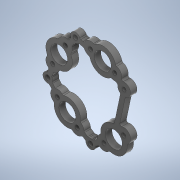
# Autodesk Inventor part: アーム モーターマウントフレーム
Saved by Autodesk Inventor 2020.2 (Build 242310000, 310)
## iProperties
Created: 2020-05-03
Part Number: アーム モーターマウントフレーム
Material: ABS プラスチック
Document SubType Name: Modeling
Designer: mozar
Density: 1.06 g/cm^3
Appearance: 滑らか - 黒
Mass: 3.91189 g
Surface Area: 42.0198 cm^2
Volume: 3.69046 cm^3
Author: mozar
Autodesk Inventor part; units mm, degrees
(part 1 of 2)
ref_plane "YZ Plane" through (0, 0, 0) normal (1, 0, 0) x (0, 1, 0)
ref_plane "XZ Plane" through (0, 0, 0) normal (0, 1, 0) x (-1, 0, 0)
ref_plane "XY Plane" through (0, 0, 0) normal (0, 0, 1) x (1, 0, 0)
sketch "スケッチ1" plane through (0, 0, 0) normal (0, 0, 1) x (1, 0, 0)
  circle A0 centre (-44.5012, 92.4909) radius 1.25
  arc A1 (-69.4548, 57.7196) -> (-69.0181, 56.9729) centre (-68.4582, 57.8015) ccw
  line L0 (-69.0181, 56.9729) -> (-68.4366, 56.58)
  arc A2 (-68.4366, 56.58) -> (-66.8767, 57.4086) centre (-67.8767, 57.4086) ccw
  line L1 (-66.8767, 57.4086) -> (-66.8767, 71.7112)
  arc A3 (-66.8767, 71.7112) -> (-67.5826, 72.667) centre (-67.8767, 71.7112) ccw
  arc A4 (-72.0424, 76.3973) -> (-67.5826, 72.667) centre (-65.3767, 79.8352) ccw
  arc A5 (-72.0424, 76.3973) -> (-73.1078, 76.9232) centre (-72.9311, 75.9389) ccw
  line L2 (-73.1078, 76.9232) -> (-87.1853, 74.3957)
  arc A6 (-87.1853, 74.3957) -> (-87.7252, 72.7139) centre (-87.0086, 73.4114) ccw
  line L3 (-87.7252, 72.7139) -> (-87.2357, 72.211)
  arc A7 (-87.2357, 72.211) -> (-86.4237, 71.9131) centre (-86.5192, 72.9085) ccw
  arc A8 (-83.0085, 70.7089) -> (-86.4237, 71.9131) centre (-86.0131, 67.6327) ccw
  arc A9 (-83.0085, 70.7089) -> (-82.0468, 70.4595) centre (-82.3098, 71.4243) ccw
  arc A10 (-71.659, 61.7707) -> (-82.0468, 70.4595) centre (-79.8767, 62.5) ccw
  arc A11 (-71.659, 61.7707) -> (-71.2436, 60.8681) centre (-70.663, 61.6823) ccw
  arc A12 (-69.4548, 57.7196) -> (-71.2436, 60.8681) centre (-73.7404, 57.3673) ccw
  arc A13 (-69.2468, 101.9882) -> (-69.916, 102.5363) centre (-70.1527, 101.5647) ccw
  line L4 (-69.916, 102.5363) -> (-70.5978, 102.7024)
  arc A14 (-70.5978, 102.7024) -> (-71.772, 101.383) centre (-70.8345, 101.7308) ccw
  line L5 (-71.772, 101.383) -> (-66.7965, 87.9737)
  arc A15 (-66.7965, 87.9737) -> (-65.8023, 87.3231) centre (-65.859, 88.3215) ccw
  arc A16 (-63.8426, 87.1766) -> (-65.8023, 87.3231) centre (-65.3767, 79.8352) ccw
  arc A17 (-63.8426, 87.1766) -> (-62.7626, 87.6721) centre (-63.638, 88.1555) ccw
  line L6 (-62.7626, 87.6721) -> (-60.3455, 92.0492)
  arc A18 (-60.3455, 92.0492) -> (-60.8525, 93.4623) centre (-61.2209, 92.5326) ccw
  arc A19 (-65.771, 98.9569) -> (-60.8525, 93.4623) centre (-57.8128, 101.1319) ccw
  arc A20 (-65.771, 98.9569) -> (-66.4744, 99.6586) centre (-66.7356, 98.6933) ccw
  arc A21 (-69.2468, 101.9882) -> (-66.4744, 99.6586) centre (-65.3514, 103.8094) ccw
  arc A22 (-69.9385, 85.7884) -> (-69.6092, 86.93) centre (-70.5467, 86.5822) ccw
  line L7 (-69.6092, 86.93) -> (-74.5846, 100.3393)
  arc A23 (-74.5846, 100.3393) -> (-76.3353, 100.5735) centre (-75.5222, 99.9915) ccw
  line L8 (-76.3353, 100.5735) -> (-76.7438, 100.0029)
  arc A24 (-76.7438, 100.0029) -> (-76.8935, 99.1509) centre (-75.9306, 99.4208) ccw
  arc A25 (-77.4753, 95.5768) -> (-76.8935, 99.1509) centre (-81.034, 97.9904) ccw
  arc A26 (-77.4753, 95.5768) -> (-77.5508, 94.5861) centre (-76.6477, 95.0154) ccw
  arc A27 (-84.2672, 82.8263) -> (-77.5508, 94.5861) centre (-85.0015, 91.0436) ccw
  arc A28 (-84.2672, 82.8263) -> (-85.0821, 82.2579) centre (-84.1781, 81.8303) ccw
  arc A29 (-87.865, 79.9409) -> (-85.0821, 82.2579) centre (-88.9691, 84.0968) ccw
  arc A30 (-87.865, 79.9409) -> (-88.5227, 79.3791) centre (-87.6082, 78.9744) ccw
  line L9 (-88.5227, 79.3791) -> (-88.8067, 78.7374)
  arc A31 (-88.8067, 78.7374) -> (-87.7155, 77.3484) centre (-87.8922, 78.3327) ccw
  line L10 (-87.7155, 77.3484) -> (-73.638, 79.876)
  arc A32 (-73.638, 79.876) -> (-72.822, 80.7396) centre (-73.8147, 80.8602) ccw
  arc A33 (-69.9385, 85.7884) -> (-72.822, 80.7396) centre (-65.3767, 79.8352) ccw
  arc A34 (13.5891, 109.0089) -> (14.6006, 109.7003) centre (13.6488, 110.0071) ccw
  line L11 (14.6006, 109.7003) -> (22.3119, 133.625)
  arc A35 (22.3119, 133.625) -> (21.598, 134.903) centre (21.3602, 133.9317) ccw
  arc A36 (21.598, 134.903) -> (-12.3137, 125.4554) centre (13.05, 100) ccw
  arc A37 (-12.3137, 125.4554) -> (-11.2534, 123.8119) centre (-11.6078, 124.747) ccw
  arc A38 (-5.288, 118.533) -> (-11.2534, 123.8119) centre (-9.6587, 119.604) ccw
  arc A39 (-5.288, 118.533) -> (-4.9702, 117.5381) centre (-4.3167, 118.295) ccw
  line L12 (-4.9702, 117.5381) -> (6.6814, 107.4795)
  arc A40 (6.6814, 107.4795) -> (7.905, 107.4148) centre (7.3349, 108.2364) ccw
  arc A41 (13.5891, 109.0089) -> (7.905, 107.4148) centre (13.05, 100) ccw
  arc A42 (16.2852, 90.7245) -> (15.1677, 91.227) centre (15.4023, 90.2549) ccw
  arc A43 (12.0966, 91.0255) -> (15.1677, 91.227) centre (13.05, 100) ccw
  arc A44 (12.0966, 91.0255) -> (11.0543, 90.3814) centre (11.9909, 90.0311) ccw
  line L13 (11.0543, 90.3814) -> (-1.3153, 57.3061)
  arc A45 (-1.3153, 57.3061) -> (-0.2632, 55.9625) centre (-0.3787, 56.9558) ccw
  line L14 (-0.2632, 55.9625) -> (26.3316, 59.055)
  arc A46 (26.3316, 59.055) -> (27.2024, 59.8834) centre (26.2161, 60.0483) ccw
  arc A47 (29.5215, 64.3049) -> (27.2024, 59.8834) centre (35.0928, 58.5637) ccw
  arc A48 (29.5215, 64.3049) -> (29.708, 65.4922) centre (28.8251, 65.0226) ccw
  line L15 (29.708, 65.4922) -> (16.2852, 90.7245)
  arc A49 (21.5566, 103.0147) -> (22.5876, 102.3526) centre (22.4992, 103.3487) ccw
  line L16 (22.5876, 102.3526) -> (47.6258, 104.5754)
  arc A50 (47.6258, 104.5754) -> (48.5246, 105.731) centre (47.5374, 105.5715) ccw
  arc A51 (48.5246, 105.731) -> (26.4932, 133.3253) centre (13.05, 100) ccw
  arc A52 (26.4932, 133.3253) -> (25.1673, 132.7046) centre (26.1191, 132.3979) ccw
  line L17 (25.1673, 132.7046) -> (17.4559, 108.78)
  arc A53 (17.4559, 108.78) -> (17.8733, 107.628) centre (18.4077, 108.4732) ccw
  arc A54 (21.5566, 103.0147) -> (17.8733, 107.628) centre (13.05, 100) ccw
  arc A55 (48.9794, 100.608) -> (47.8911, 101.5872) centre (47.9795, 100.5911) ccw
  line L18 (47.8911, 101.5872) -> (22.8529, 99.3644)
  arc A56 (22.8529, 99.3644) -> (21.9546, 98.5311) centre (22.9413, 98.3683) ccw
  arc A57 (19.1416, 93.341) -> (21.9546, 98.5311) centre (13.05, 100) ccw
  arc A58 (19.1416, 93.341) -> (18.9338, 92.1335) centre (19.8166, 92.6031) ccw
  line L19 (18.9338, 92.1335) -> (30.7392, 69.9415)
  arc A59 (30.7392, 69.9415) -> (32.1537, 69.5642) centre (31.622, 70.4111) ccw
  arc A60 (32.1537, 69.5642) -> (48.9794, 100.608) centre (13.05, 100) ccw
  arc A61 (-34.2364, 127.0372) -> (-36.0614, 127.7726) centre (-35.216, 127.2385) ccw
  line L20 (-36.0614, 127.7726) -> (-39.8212, 121.8216)
  arc A62 (-39.8212, 121.8216) -> (-38.4894, 120.4137) centre (-38.9758, 121.2874) ccw
  line L21 (-38.4894, 120.4137) -> (-34.6838, 122.5323)
  arc A63 (-34.6838, 122.5323) -> (-34.1958, 123.6306) centre (-35.1702, 123.406) ccw
  arc A64 (-34.2364, 127.0372) -> (-34.1958, 123.6306) centre (-26.4001, 125.4272) ccw
  arc A65 (5.9328, 94.4506) -> (4.7454, 94.7527) centre (5.1442, 93.8357) ccw
  line L22 (4.7454, 94.7527) -> (-16.5104, 85.5088)
  arc A66 (-16.5104, 85.5088) -> (-17.0899, 84.3844) centre (-16.1116, 84.5918) ccw
  arc A67 (-19.2338, 74.9766) -> (-17.0899, 84.3844) centre (-28.3399, 82) ccw
  arc A68 (-19.2338, 74.9766) -> (-19.1987, 73.7122) centre (-18.4419, 74.3659) ccw
  line L23 (-19.1987, 73.7122) -> (-5.7745, 58.1716)
  arc A69 (-5.7745, 58.1716) -> (-4.0811, 58.475) centre (-5.0177, 58.8253) ccw
  line L24 (-4.0811, 58.475) -> (8.2443, 91.4322)
  arc A70 (8.2443, 91.4322) -> (7.8805, 92.6022) centre (7.3077, 91.7825) ccw
  arc A71 (5.9328, 94.4506) -> (7.8805, 92.6022) centre (13.05, 100) ccw
  arc A72 (4.9636, 104.0076) -> (4.721, 105.2086) centre (4.0676, 104.4516) ccw
  line L25 (4.721, 105.2086) -> (-6.9306, 115.2672)
  arc A73 (-6.9306, 115.2672) -> (-7.9613, 115.4364) centre (-7.5841, 114.5103) ccw
  arc A74 (-9.6102, 115.1042) -> (-7.9613, 115.4364) centre (-9.6587, 119.604) ccw
  arc A75 (-9.6102, 115.1042) -> (-10.495, 114.5492) centre (-9.5994, 114.1043) ccw
  line L26 (-10.495, 114.5492) -> (-21.5476, 92.3011)
  arc A76 (-21.5476, 92.3011) -> (-21.267, 91.0677) centre (-20.652, 91.8562) ccw
  arc A77 (-18.9244, 88.6028) -> (-21.267, 91.0677) centre (-28.3399, 82) ccw
  arc A78 (-18.9244, 88.6028) -> (-17.7068, 88.2599) centre (-18.1056, 89.177) ccw
  line L27 (-17.7068, 88.2599) -> (3.549, 97.5038)
  arc A79 (3.549, 97.5038) -> (4.1377, 98.5784) centre (3.1501, 98.4209) ccw
  arc A80 (4.9636, 104.0076) -> (4.1377, 98.5784) centre (13.05, 100) ccw
  arc A81 (-35.8272, 90.7287) -> (-35.6044, 91.9739) centre (-36.4783, 91.4878) ccw
  line L28 (-35.6044, 91.9739) -> (-45.4441, 109.6631)
  arc A82 (-45.4441, 109.6631) -> (-47.1934, 109.6604) centre (-46.318, 109.177) ccw
  line L29 (-47.1934, 109.6604) -> (-49.9541, 104.6611)
  arc A83 (-49.9541, 104.6611) -> (-50.0229, 103.8484) centre (-49.0787, 104.1777) ccw
  arc A84 (-49.8547, 103.3068) -> (-50.0229, 103.8484) centre (-57.8128, 101.1319) ccw
  arc A85 (-49.8547, 103.3068) -> (-49.1512, 102.6051) centre (-48.89, 103.5704) ccw
  arc A86 (-46.0508, 97.6465) -> (-49.1512, 102.6051) centre (-50.2742, 98.4544) ccw
  arc A87 (-46.0508, 97.6465) -> (-44.9551, 96.465) centre (-45.0686, 97.4586) ccw
  arc A88 (-40.5067, 92.2823) -> (-44.9551, 96.465) centre (-44.5012, 92.4909) ccw
  arc A89 (-40.5067, 92.2823) -> (-40.0525, 91.3914) centre (-39.5081, 92.2301) ccw
  line L30 (-40.0525, 91.3914) -> (-37.7961, 89.9266)
  arc A90 (-37.7961, 89.9266) -> (-36.5387, 90.0642) centre (-37.2516, 90.7654) ccw
  arc A91 (-35.8272, 90.7287) -> (-36.5387, 90.0642) centre (-28.3399, 82) ccw
  arc A92 (-35.3558, 72.8881) -> (-36.6202, 72.8519) centre (-35.9659, 72.0957) ccw
  line L31 (-36.6202, 72.8519) -> (-40.2601, 69.7025)
  arc A93 (-40.2601, 69.7025) -> (-40.5745, 68.6985) centre (-39.6057, 68.9463) ccw
  arc A94 (-42.2436, 64.1319) -> (-40.5745, 68.6985) centre (-44.7404, 67.6327) ccw
  arc A95 (-42.2436, 64.1319) -> (-42.659, 63.2293) centre (-41.663, 63.3177) ccw
  arc A96 (-50.0378, 54.2928) -> (-42.659, 63.2293) centre (-50.8767, 62.5) ccw
  arc A97 (-50.0378, 54.2928) -> (-50.8242, 52.8384) centre (-49.9361, 53.298) ccw
  arc A98 (-50.7048, 52.5865) -> (-50.8242, 52.8384) centre (-54.3767, 51) ccw
  arc A99 (-50.7048, 52.5865) -> (-49.7048, 51.9865) centre (-49.7868, 52.9832) ccw
  arc A100 (-46.9767, 51.2) -> (-49.7048, 51.9865) centre (-49.3767, 48) ccw
  arc A101 (-46.9767, 51.2) -> (-46.3767, 51) centre (-46.3767, 52) ccw
  line L32 (-46.3767, 51) -> (-7.6173, 51)
  arc A102 (-7.6173, 51) -> (-6.7512, 52.5) centre (-7.6173, 52) ccw
  arc A103 (-7.103, 54.5465) -> (-6.7512, 52.5) centre (-4.1532, 54) ccw
  arc A104 (-7.103, 54.5465) -> (-7.3295, 55.3824) centre (-8.0862, 54.7287) ccw
  line L33 (-7.3295, 55.3824) -> (-21.469, 71.7511)
  arc A105 (-21.469, 71.7511) -> (-22.7149, 71.9696) centre (-22.2257, 71.0974) ccw
  arc A106 (-35.3558, 72.8881) -> (-22.7149, 71.9696) centre (-28.3399, 82) ccw
  arc A107 (-43.3166, 71.6902) -> (-42.3312, 71.8776) centre (-42.9855, 72.6338) ccw
  line L34 (-42.3312, 71.8776) -> (-38.5832, 75.1206)
  arc A108 (-38.5832, 75.1206) -> (-38.3657, 76.3667) centre (-39.2375, 75.8768) ccw
  arc A109 (-39.4542, 79.0465) -> (-38.3657, 76.3667) centre (-28.3399, 82) ccw
  arc A110 (-39.4542, 79.0465) -> (-40.479, 79.7879) centre (-40.4207, 78.7896) ccw
  line L35 (-40.479, 79.7879) -> (-57.179, 78.8118)
  arc A111 (-57.179, 78.8118) -> (-58.092, 78.0514) centre (-57.1207, 77.8135) ccw
  arc A112 (-63.1709, 72.667) -> (-58.092, 78.0514) centre (-65.3767, 79.8352) ccw
  arc A113 (-63.1709, 72.667) -> (-63.8767, 71.7112) centre (-62.8767, 71.7112) ccw
  line L36 (-63.8767, 71.7112) -> (-63.8767, 57.4086)
  arc A114 (-63.8767, 57.4086) -> (-62.3169, 56.58) centre (-62.8767, 57.4086) ccw
  line L37 (-62.3169, 56.58) -> (-61.7354, 56.9729)
  arc A115 (-61.7354, 56.9729) -> (-61.2986, 57.7196) centre (-62.2953, 57.8015) ccw
  arc A116 (-59.5099, 60.8681) -> (-61.2986, 57.7196) centre (-57.0131, 57.3673) ccw
  arc A117 (-59.5099, 60.8681) -> (-59.0944, 61.7707) centre (-60.0905, 61.6823) ccw
  arc A118 (-48.7067, 70.4595) -> (-59.0944, 61.7707) centre (-50.8767, 62.5) ccw
  arc A119 (-48.7067, 70.4595) -> (-47.7449, 70.7089) centre (-48.4437, 71.4243) ccw
  arc A120 (-43.3166, 71.6902) -> (-47.7449, 70.7089) centre (-44.7404, 67.6327) ccw
  arc A121 (-24.5231, 117.6505) -> (-25.2874, 116.723) centre (-24.2884, 116.6784) ccw
  line L38 (-25.2874, 116.723) -> (-26.2949, 94.1683)
  arc A122 (-26.2949, 94.1683) -> (-25.5394, 93.1538) centre (-25.2959, 94.1237) ccw
  arc A123 (-25.3867, 93.1143) -> (-25.5394, 93.1538) centre (-28.3399, 82) ccw
  arc A124 (-25.3867, 93.1143) -> (-24.2343, 93.6359) centre (-25.1298, 94.0808) ccw
  line L39 (-24.2343, 93.6359) -> (-13.1817, 115.8839)
  arc A125 (-13.1817, 115.8839) -> (-13.2739, 116.9243) centre (-14.0773, 116.3288) ccw
  arc A126 (-14.1165, 118.9889) -> (-13.2739, 116.9243) centre (-9.6587, 119.604) ccw
  arc A127 (-14.1165, 118.9889) -> (-14.7786, 119.7967) centre (-15.1071, 118.8522) ccw
  line L40 (-14.7786, 119.7967) -> (-18.727, 121.17)
  arc A128 (-18.727, 121.17) -> (-19.8716, 120.8035) centre (-19.0555, 120.2256) ccw
  arc A129 (-24.5231, 117.6505) -> (-19.8716, 120.8035) centre (-26.4001, 125.4272) ccw
  arc A130 (-30.1348, 93.3591) -> (-29.2919, 94.3022) centre (-30.2909, 94.3468) ccw
  line L41 (-29.2919, 94.3022) -> (-28.2844, 116.8569)
  arc A131 (-28.2844, 116.8569) -> (-28.9631, 117.8488) centre (-29.2834, 116.9015) ccw
  arc A132 (-32.0339, 119.7474) -> (-28.9631, 117.8488) centre (-26.4001, 125.4272) ccw
  arc A133 (-32.0339, 119.7474) -> (-33.2246, 119.9111) centre (-32.7382, 119.0374) ccw
  line L42 (-33.2246, 119.9111) -> (-42.8681, 114.5425)
  arc A134 (-42.8681, 114.5425) -> (-43.3678, 113.8351) centre (-42.3817, 113.6687) ccw
  arc A135 (-43.549, 113.1991) -> (-43.3678, 113.8351) centre (-46.326, 114.3342) ccw
  arc A136 (-43.549, 113.1991) -> (-43.4972, 112.3347) centre (-42.6234, 112.8208) ccw
  line L43 (-43.4972, 112.3347) -> (-32.9827, 93.4322)
  arc A137 (-32.9827, 93.4322) -> (-31.8073, 92.9648) centre (-32.1088, 93.9183) ccw
  arc A138 (-30.1348, 93.3591) -> (-31.8073, 92.9648) centre (-28.3399, 82) ccw
  arc A139 (-39.0433, 86.2058) -> (-39.4295, 87.4103) centre (-39.974, 86.5715) ccw
  line L44 (-39.4295, 87.4103) -> (-41.686, 88.875)
  arc A140 (-41.686, 88.875) -> (-42.6846, 88.9272) centre (-42.2304, 88.0363) ccw
  arc A141 (-48.4958, 92.6994) -> (-42.6846, 88.9272) centre (-44.5012, 92.4909) ccw
  arc A142 (-48.4958, 92.6994) -> (-48.95, 93.5904) centre (-49.4944, 92.7516) ccw
  line L45 (-48.95, 93.5904) -> (-49.574, 93.9954)
  arc A143 (-49.574, 93.9954) -> (-50.1478, 94.1562) centre (-50.1185, 93.1567) ccw
  arc A144 (-52.021, 94.5252) -> (-50.1478, 94.1562) centre (-50.2742, 98.4544) ccw
  arc A145 (-52.021, 94.5252) -> (-53.0094, 94.4244) centre (-52.4272, 93.6114) ccw
  arc A146 (-55.9627, 93.092) -> (-53.0094, 94.4244) centre (-57.8128, 101.1319) ccw
  arc A147 (-55.9627, 93.092) -> (-56.6139, 92.6009) centre (-55.7385, 92.1174) ccw
  line L46 (-56.6139, 92.6009) -> (-60.1364, 86.2219)
  arc A148 (-60.1364, 86.2219) -> (-59.9805, 85.044) centre (-59.261, 85.7385) ccw
  arc A149 (-58.3494, 82.4556) -> (-59.9805, 85.044) centre (-65.3767, 79.8352) ccw
  arc A150 (-58.3494, 82.4556) -> (-57.3541, 81.8067) centre (-57.4124, 82.805) ccw
  line L47 (-57.3541, 81.8067) -> (-40.6541, 82.7828)
  arc A151 (-40.6541, 82.7828) -> (-39.7226, 83.6386) centre (-40.7124, 83.7811) ccw
  arc A152 (-39.0433, 86.2058) -> (-39.7226, 83.6386) centre (-28.3399, 82) ccw
  arc A153 (-76.6906, 54.239) -> (-78.3767, 53.5115) centre (-77.3767, 53.5115) ccw
  line L48 (-78.3767, 53.5115) -> (-78.3767, 52)
  arc A154 (-78.3767, 52) -> (-77.3767, 51) centre (-77.3767, 52) ccw
  line L49 (-77.3767, 51) -> (-69.3767, 51)
  arc A155 (-69.3767, 51) -> (-68.7767, 51.2) centre (-69.3767, 52) ccw
  arc A156 (-68.7327, 51.2326) -> (-68.7767, 51.2) centre (-66.3767, 48) ccw
  arc A157 (-68.7327, 51.2326) -> (-68.3354, 52.206) centre (-69.3217, 52.0407) ccw
  arc A158 (-68.3669, 52.4596) -> (-68.3354, 52.206) centre (-65.3767, 52.702) ccw
  arc A159 (-68.3669, 52.4596) -> (-68.8038, 53.2074) centre (-69.3637, 52.3788) ccw
  line L50 (-68.8038, 53.2074) -> (-69.9585, 53.9877)
  arc A160 (-69.9585, 53.9877) -> (-71.1263, 53.9531) centre (-70.5184, 53.1591) ccw
  arc A161 (-76.6906, 54.239) -> (-71.1263, 53.9531) centre (-73.7404, 57.3673) ccw
  arc A162 (23.6969, 52.5865) -> (24.6969, 51.9865) centre (24.6149, 52.9832) ccw
  arc A163 (27.425, 51.2) -> (24.6969, 51.9865) centre (25.025, 48) ccw
  arc A164 (27.425, 51.2) -> (28.025, 51) centre (28.025, 52) ccw
  line L51 (28.025, 51) -> (28.935, 51)
  arc A165 (28.935, 51) -> (29.6192, 52.7293) centre (28.935, 52) ccw
  arc A166 (27.7157, 55.4687) -> (29.6192, 52.7293) centre (35.0928, 58.5637) ccw
  arc A167 (27.7157, 55.4687) -> (26.6781, 56.0751) centre (26.7936, 55.0818) ccw
  line L52 (26.6781, 56.0751) -> (23.2864, 55.6807)
  arc A168 (23.2864, 55.6807) -> (22.7265, 53.9499) centre (23.4019, 54.6874) ccw
  arc A169 (23.6969, 52.5865) -> (22.7265, 53.9499) centre (20.025, 51) ccw
  arc A170 (5.025, 51) -> (5.625, 51.2) centre (5.025, 52) ccw
  arc A171 (8.3531, 51.9865) -> (5.625, 51.2) centre (8.025, 48) ccw
  arc A172 (8.3531, 51.9865) -> (7.8023, 53.8801) centre (7.9178, 52.8868) ccw
  line L53 (7.8023, 53.8801) -> (0.176, 52.9933)
  arc A173 (0.176, 52.9933) -> (0.2915, 51) centre (0.2915, 52) ccw
  line L54 (0.2915, 51) -> (5.025, 51)
  arc A174 (-48.3767, 48) -> (-50.3767, 48) centre (-49.3767, 48) ccw
  line L55 (-50.3767, 48) -> (-50.3767, 45)
  line L56 (-50.3767, 45) -> (-65.3767, 45)
  line L57 (-65.3767, 45) -> (-65.3767, 48)
  arc A175 (-65.3767, 48) -> (-67.3767, 48) centre (-66.3767, 48) ccw
  line L58 (-67.3767, 48) -> (-81.3767, 48)
  line L59 (-81.3767, 48) -> (-81.3767, 53.5942)
  arc A176 (-81.3767, 53.5942) -> (-82.1065, 54.557) centre (-82.3767, 53.5942) ccw
  arc A177 (-88.0944, 63.2293) -> (-82.1065, 54.557) centre (-79.8767, 62.5) ccw
  arc A178 (-88.0944, 63.2293) -> (-88.5099, 64.1319) centre (-89.0905, 63.3177) ccw
  arc A179 (-89.8355, 69.6024) -> (-88.5099, 64.1319) centre (-86.0131, 67.6327) ccw
  arc A180 (-89.8355, 69.6024) -> (-90.0078, 70.7579) centre (-90.7244, 70.0604) ccw
  line L60 (-90.0078, 70.7579) -> (-90.9798, 71.7565)
  arc A181 (-90.9798, 71.7565) -> (-91.7931, 72.0544) centre (-91.6964, 71.059) ccw
  arc A182 (-92.8499, 77.9406) -> (-91.7931, 72.0544) centre (-92.0829, 75.0403) ccw
  arc A183 (-92.8499, 77.9406) -> (-92.1911, 78.5027) centre (-93.1056, 78.9074) ccw
  line L61 (-92.1911, 78.5027) -> (-91.6272, 79.7771)
  arc A184 (-91.6272, 79.7771) -> (-91.8676, 80.9205) centre (-92.5416, 80.1818) ccw
  arc A185 (-92.5278, 86.5104) -> (-91.8676, 80.9205) centre (-88.9691, 84.0968) ccw
  arc A186 (-92.5278, 86.5104) -> (-92.4523, 87.5011) centre (-93.3554, 87.0717) ccw
  arc A187 (-85.7359, 99.2608) -> (-92.4523, 87.5011) centre (-85.0015, 91.0436) ccw
  arc A188 (-85.7359, 99.2608) -> (-84.921, 99.8292) centre (-85.8249, 100.2569) ccw
  arc A189 (-79.7708, 102.1007) -> (-84.921, 99.8292) centre (-81.034, 97.9904) ccw
  arc A190 (-79.7708, 102.1007) -> (-78.6639, 102.4745) centre (-79.4771, 103.0566) ccw
  line L62 (-78.6639, 102.4745) -> (-77.8528, 103.6077)
  arc A191 (-77.8528, 103.6077) -> (-77.7034, 104.4608) centre (-78.6659, 104.1898) ccw
  arc A192 (-72.0965, 106.5412) -> (-77.7034, 104.4608) centre (-74.8156, 105.2737) ccw
  arc A193 (-72.0965, 106.5412) -> (-71.4268, 105.9921) centre (-71.1901, 106.9637) ccw
  line L63 (-71.4268, 105.9921) -> (-70.0728, 105.6623)
  arc A194 (-70.0728, 105.6623) -> (-68.99, 106.1009) centre (-69.8361, 106.6338) ccw
  arc A195 (-63.6047, 107.7386) -> (-68.99, 106.1009) centre (-65.3514, 103.8094) ccw
  arc A196 (-63.6047, 107.7386) -> (-62.6162, 107.8393) centre (-63.1984, 108.6523) ccw
  arc A197 (-52.9408, 107.7896) -> (-62.6162, 107.8393) centre (-57.8128, 101.1319) ccw
  arc A198 (-52.9408, 107.7896) -> (-51.4748, 108.1132) centre (-52.3502, 108.5966) ccw
  line L64 (-51.4748, 108.1132) -> (-49.1485, 112.3259)
  arc A199 (-49.1485, 112.3259) -> (-49.0994, 113.1906) centre (-50.0239, 112.8093) ccw
  arc A200 (-46.6603, 117.3156) -> (-49.0994, 113.1906) centre (-46.326, 114.3342) ccw
  arc A201 (-46.6603, 117.3156) -> (-45.9263, 117.7752) centre (-46.7717, 118.3093) ccw
  line L65 (-45.9263, 117.7752) -> (-37.8629, 130.5378)
  arc A202 (-37.8629, 130.5378) -> (-37.763, 131.3981) centre (-38.7083, 131.0719) ccw
  arc A203 (-31.9852, 132.9642) -> (-37.763, 131.3981) centre (-34.927, 132.3764) ccw
  arc A204 (-31.9852, 132.9642) -> (-30.493, 132.3009) centre (-31.0046, 133.1602) ccw
  arc A205 (-18.408, 125.7823) -> (-30.493, 132.3009) centre (-26.4001, 125.4272) ccw
  arc A206 (-18.408, 125.7823) -> (-16.6463, 125.18) centre (-17.409, 125.8267) ccw
  arc A207 (35.6612, 68.3041) -> (-16.6463, 125.18) centre (13.05, 100) ccw
  arc A208 (35.6612, 68.3041) -> (36.1143, 66.4982) centre (36.242, 67.49) ccw
  arc A209 (42.206, 54.9028) -> (36.1143, 66.4982) centre (35.0928, 58.5637) ccw
  arc A210 (42.206, 54.9028) -> (42.9601, 53.4544) centre (43.0951, 54.4452) ccw
  arc A211 (41.0782, 47.8705) -> (42.9601, 53.4544) centre (42.5549, 50.4818) ccw
  arc A212 (41.0782, 47.8705) -> (40.586, 48) centre (40.586, 47) ccw
  line L66 (40.586, 48) -> (26.025, 48)
  arc A213 (26.025, 48) -> (24.025, 48) centre (25.025, 48) ccw
  line L67 (24.025, 48) -> (24.025, 45)
  line L68 (24.025, 45) -> (9.025, 45)
  line L69 (9.025, 45) -> (9.025, 48)
  arc A214 (9.025, 48) -> (7.025, 48) centre (8.025, 48) ccw
  line L70 (7.025, 48) -> (-48.3767, 48)
  arc A215 (-55.3767, 48) -> (-53.3767, 48) centre (-54.3767, 48) ccw
  line L71 (-53.3767, 48) -> (-53.3767, 51)
  arc A216 (-53.3767, 51) -> (-55.3767, 51) centre (-54.3767, 51) ccw
  line L72 (-55.3767, 51) -> (-60.3767, 51)
  arc A217 (-60.3767, 51) -> (-62.3767, 51) centre (-61.3767, 51) ccw
  line L73 (-62.3767, 51) -> (-62.3767, 48)
  arc A218 (-62.3767, 48) -> (-60.3767, 48) centre (-61.3767, 48) ccw
  line L74 (-60.3767, 48) -> (-55.3767, 48)
  arc A219 (12.025, 48) -> (14.025, 48) centre (13.025, 48) ccw
  line L75 (14.025, 48) -> (19.025, 48)
  arc A220 (19.025, 48) -> (21.025, 48) centre (20.025, 48) ccw
  line L76 (21.025, 48) -> (21.025, 51)
  arc A221 (21.025, 51) -> (19.025, 51) centre (20.025, 51) ccw
  line L77 (19.025, 51) -> (14.025, 51)
  arc A222 (14.025, 51) -> (12.025, 51) centre (13.025, 51) ccw
  line L78 (12.025, 51) -> (12.025, 48)
  circle A223 centre (-4.1532, 54) radius 1.5
  circle A224 centre (-46.326, 114.3342) radius 1.5
  circle A225 centre (-34.927, 132.3764) radius 1.5
  circle A226 centre (42.5549, 50.4818) radius 1.5
  circle A227 centre (-26.4001, 125.4272) radius 4
  circle A228 centre (35.0928, 58.5637) radius 4
  circle A229 centre (-74.8156, 105.2737) radius 1.5
  circle A230 centre (-65.3767, 52.702) radius 1.5
  circle A231 centre (-44.7404, 67.6327) radius 1.3
  circle A232 centre (-57.0131, 57.3673) radius 1.3
  circle A233 centre (-50.8767, 62.5) radius 5.25
  circle A234 centre (-92.0829, 75.0403) radius 1.5
  circle A235 centre (-65.3767, 79.8352) radius 4.5
  circle A236 centre (-28.3399, 82) radius 7.5
  circle A237 centre (-73.7404, 57.3673) radius 1.3
  circle A238 centre (-86.0131, 67.6327) radius 1.3
  circle A239 centre (-79.8767, 62.5) radius 5.25
  circle A240 centre (-65.3514, 103.8094) radius 1.3
  circle A241 centre (-50.2742, 98.4544) radius 1.3
  circle A242 centre (-57.8128, 101.1319) radius 5.25
  circle A243 centre (-9.6587, 119.604) radius 1.5
  circle A244 centre (13.05, 100) radius 4.025
  circle A245 centre (-88.9691, 84.0968) radius 1.3
  circle A246 centre (-81.034, 97.9904) radius 1.3
  circle A247 centre (-85.0015, 91.0436) radius 5.25
  line L79 (-50.8767, 62.5) -> (-44.5012, 92.4909) construction
  line L80 (-49.4095, 62.1881) -> (-43.034, 92.179)
  line L81 (-45.9685, 92.8028) -> (-52.344, 62.8119)
  arc A248 (-52.344, 62.8119) -> (-49.4095, 62.1881) centre (-50.8767, 62.5) ccw
  arc A249 (-43.034, 92.179) -> (-45.9685, 92.8028) centre (-44.5012, 92.4909) ccw
  circle A250 centre (-65.3767, 79.8352) radius 7.5
  circle A251 centre (-57.8128, 101.1319) radius 8.25
  line L82 (-65.3767, 79.8352) -> (-44.5012, 92.4909) construction
  line L83 (-64.5991, 78.5525) -> (-43.7236, 91.2082)
  line L84 (-45.2789, 93.7736) -> (-66.1544, 81.1179)
  arc A252 (-66.1544, 81.1179) -> (-64.5991, 78.5525) centre (-65.3767, 79.8352) ccw
  arc A253 (-43.7236, 91.2082) -> (-45.2789, 93.7736) centre (-44.5012, 92.4909) ccw
  circle A254 centre (-79.8767, 62.5) radius 8.25
  circle A255 centre (-65.3767, 52.702) radius 3
  line L85 (-65.3767, 52.702) -> (-50.8767, 62.5) construction
  line L86 (-64.5369, 51.4592) -> (-50.0369, 61.2571)
  line L87 (-51.7166, 63.7429) -> (-66.2166, 53.9449)
  arc A256 (-66.2166, 53.9449) -> (-64.5369, 51.4592) centre (-65.3767, 52.702) ccw
  arc A257 (-50.0369, 61.2571) -> (-51.7166, 63.7429) centre (-50.8767, 62.5) ccw
  circle A258 centre (-57.0131, 57.3673) radius 4.3
  circle A259 centre (-50.8767, 62.5) radius 8.25
  circle A260 centre (-44.7404, 67.6327) radius 4.3
  circle A261 centre (-44.5012, 92.4909) radius 4
  circle A262 centre (-73.7404, 57.3673) radius 4.3
  point P0 (0, 0)
  point P1 (0, 0)
  point P2 (-47.689, 77.4954)
  point P3 (-54.939, 86.163)
  point P4 (-58.1267, 57.601)
  point P5 (-59.8705, 84.9275)
  point P6 (-59.9805, 85.044)
  point P7 (-48.4498, 91.8512)
  point P8 (-58.3104, 82.365)
  point P9 (-46.8945, 89.2858)
  point P10 (-46.7395, 89.1757)
  point P11 (-50.6571, 70.7471)
  point P12 (-59.0189, 61.1708)
  point P13 (-61.3117, 57.2592)
  point P14 (-64.0639, 55.3995)
  point P15 (-62.3842, 52.9138)
  point P16 (-60.1485, 54.4246)
  point P17 (-53.6239, 54.7208)
  point P18 (-42.659, 63.2293)
  point P19 (-42.7345, 63.8292)
  point P20 (-47.5624, 70.8772)
  point P21 (-43.8051, 88.5519)
  point P22 (-42.6846, 88.9272)
  point P23 (-50.0229, 103.8484)
  point P24 (-74.4553, 56.2815)
  point P25 (-72.798, 58.2628)
  point P26 (-67.5826, 72.667)
  point P27 (-58.092, 78.0514)
  point P28 (-77.1295, 54.7208)
  point P29 (-67.5826, 72.667)
  point P30 (-71.7345, 61.1708)
  dimension "d0" = 3
  dimension "d1" = 3
  dimension "d2" = 3
  constraints: 456 point on circle, 255 centre point, 182 end point, 13 horizontal, 12 tangent, 12 vertical, 9 coincident, 3 concentric, 3 midpoint, 3 parallel, 877 other
  measures "d0" diameter of A249
  measures "d1" diameter of A253
  measures "d2" diameter of A257
extrude "押し出し1" add sketch "スケッチ1" against normal blind 4 contours A262 A161 A254 A237 A12 | A1 L0 A2 L1 A3 A250 A113 L36 A114 L87 A255 A159 L50 A160 A262 | A254 A262 A239 A177 A238 A10 | A254 A237 A262 A239 | A254 A238 A178 A179 A180 L60 A181 A182 A183 L61 A184 A185 A186 A187 A188 A189 A190 L62 A191 A192 A193 L63 A194 A195 A196 A251 A240 A20 A21 A13 L4 A14 L5 A15 A250 A22 L7 A23 L8 A24 A25 A26 A27 A28 A29 A30 L9 A31 L10 A32 A5 L2 A6 L3 A7 A8 A9 | A4 A250 A33 A16 A149 L84 A235 L83 A112 | A255 L87 A230 L86 A158 | L87 L37 A258 L86 A255 | A255 L86 A230 L87 | A258 L87 A259 A232 L86 | L86 A232 A259 A258 | L81 L47 L80 L35 | L35 L80 A120 A119 A118 L81 | L83 A235 L84 A149 A150 | A150 A149 L84 A141 L83 | A258 A116 A259 L87 | A259 A232 L86 A233 A258 | A258 A233 A260 A259 A96 | L81 A141 L80 L47 | L81 A233 A258 A259 A118 | A118 A259 A260 A233 L81 | L83 L81 A141 | A141 L84 A249 L81 L83 | A259 L87 A233 L86 A232 | A259 A258 A233 L87 | L80 A259 A260 A120 | A120 A260 A94 A259 A231 L80 | L81 L83 A253 L80 A141 | A119 A260 A259 | A141 A261 A88 L80 A249 L84 | L81 A249 A253 L83 | A259 A231 A260 A233 L80 | L80 A233 A260 A259 | A142 L45 A143 A144 A145 A251 A241 A85 A86 A87 A261 | A19 A251 A240 A197 A84 A241 A146
fillet "フィレット1" radius 1 15 edges at (-46.8945, 89.2858, -2) (-46.7395, 89.1757, -2) (-50.6571, 70.7471, -2) (-59.0189, 61.1708, -2) (-61.3117, 57.2592, -2) (-71.7345, 61.1708, -2) (-62.3842, 52.9138, -2) (-77.1295, 54.7208, -2) (-60.1485, 54.4246, -2) (-53.6239, 54.7208, -2) (-42.7345, 63.8292, -2) (-47.5624, 70.8772, -2) (-43.8051, 88.5519, -2) (-59.8705, 84.9275, -2) (-48.4498, 91.8512, -2)
sketch "スケッチ2" plane through (0, 0, 0) normal (0, 0, 1) x (1, 0, 0)
  arc A0 (-83.0085, 70.7089) -> (-82.0468, 70.4595) centre (-82.3098, 71.4243) ccw projected
  arc A1 (-71.659, 61.7707) -> (-82.0468, 70.4595) centre (-79.8767, 62.5) ccw projected
  arc A2 (-71.659, 61.7707) -> (-71.2436, 60.8681) centre (-70.663, 61.6823) ccw projected
  arc A3 (-69.4548, 57.7196) -> (-71.2436, 60.8681) centre (-73.7404, 57.3673) ccw projected
  arc A4 (-69.4548, 57.7196) -> (-69.0181, 56.9729) centre (-68.4582, 57.8015) ccw projected
  line L0 (-69.0181, 56.9729) -> (-68.4366, 56.58) projected
  arc A5 (-68.4366, 56.58) -> (-66.8767, 57.4086) centre (-67.8767, 57.4086) ccw projected
  line L1 (-66.8767, 57.4086) -> (-66.8767, 71.7112) projected
  arc A6 (-66.8767, 71.7112) -> (-67.5826, 72.667) centre (-67.8767, 71.7112) ccw projected
  arc A7 (-72.0424, 76.3973) -> (-67.5826, 72.667) centre (-65.3767, 79.8352) ccw projected
  arc A8 (-72.0424, 76.3973) -> (-73.1078, 76.9232) centre (-72.9311, 75.9389) ccw projected
  line L2 (-73.1078, 76.9232) -> (-87.1853, 74.3957) projected
  arc A9 (-87.1853, 74.3957) -> (-87.7252, 72.7139) centre (-87.0086, 73.4114) ccw projected
  line L3 (-87.7252, 72.7139) -> (-87.2357, 72.211) projected
  arc A10 (-87.2357, 72.211) -> (-86.4237, 71.9131) centre (-86.5192, 72.9085) ccw projected
  arc A11 (-83.0085, 70.7089) -> (-86.4237, 71.9131) centre (-86.0131, 67.6327) ccw projected
  circle A12 centre (-73.7404, 57.3673) radius 1.3 projected
  circle A13 centre (-65.3767, 79.8352) radius 4.5 projected
  circle A14 centre (-74.8156, 105.2737) radius 1.5 projected
  circle A15 centre (-92.0829, 75.0403) radius 1.5 projected
  circle A16 centre (-85.0015, 91.0436) radius 5.25 projected
  circle A17 centre (-88.9691, 84.0968) radius 1.3 projected
  circle A18 centre (-81.034, 97.9904) radius 1.3 projected
  circle A19 centre (-65.3514, 103.8094) radius 1.3 projected
  circle A20 centre (-50.2742, 98.4544) radius 1.3 projected
  circle A21 centre (-57.8128, 101.1319) radius 5.25 projected
  circle A22 centre (-86.0131, 67.6327) radius 1.3 projected
  circle A23 centre (-79.8767, 62.5) radius 5.25 projected
  arc A24 (-73.638, 79.876) -> (-72.822, 80.7396) centre (-73.8147, 80.8602) ccw projected
  arc A25 (-69.9385, 85.7884) -> (-72.822, 80.7396) centre (-65.3767, 79.8352) ccw projected
  arc A26 (-69.9385, 85.7884) -> (-69.6092, 86.93) centre (-70.5467, 86.5822) ccw projected
  line L4 (-69.6092, 86.93) -> (-74.5846, 100.3393) projected
  arc A27 (-74.5846, 100.3393) -> (-76.3353, 100.5735) centre (-75.5222, 99.9915) ccw projected
  line L5 (-76.3353, 100.5735) -> (-76.7438, 100.0029) projected
  arc A28 (-76.7438, 100.0029) -> (-76.8935, 99.1509) centre (-75.9306, 99.4208) ccw projected
  arc A29 (-77.4753, 95.5768) -> (-76.8935, 99.1509) centre (-81.034, 97.9904) ccw projected
  arc A30 (-77.4753, 95.5768) -> (-77.5508, 94.5861) centre (-76.6477, 95.0154) ccw projected
  arc A31 (-84.2672, 82.8263) -> (-77.5508, 94.5861) centre (-85.0015, 91.0436) ccw projected
  arc A32 (-84.2672, 82.8263) -> (-85.0821, 82.2579) centre (-84.1781, 81.8303) ccw projected
  arc A33 (-87.865, 79.9409) -> (-85.0821, 82.2579) centre (-88.9691, 84.0968) ccw projected
  arc A34 (-87.865, 79.9409) -> (-88.5227, 79.3791) centre (-87.6082, 78.9744) ccw projected
  line L6 (-88.5227, 79.3791) -> (-88.8067, 78.7374) projected
  arc A35 (-88.8067, 78.7374) -> (-87.7155, 77.3484) centre (-87.8922, 78.3327) ccw projected
  line L7 (-87.7155, 77.3484) -> (-73.638, 79.876) projected
  circle A36 centre (-44.5012, 92.4909) radius 1.25 projected
  arc A37 (-69.2468, 101.9882) -> (-66.4744, 99.6586) centre (-65.3514, 103.8094) ccw projected
  arc A38 (-69.2468, 101.9882) -> (-69.916, 102.5363) centre (-70.1527, 101.5647) ccw projected
  line L8 (-69.916, 102.5363) -> (-70.5978, 102.7024) projected
  arc A39 (-70.5978, 102.7024) -> (-71.772, 101.383) centre (-70.8345, 101.7308) ccw projected
  line L9 (-71.772, 101.383) -> (-66.7965, 87.9737) projected
  arc A40 (-66.7965, 87.9737) -> (-65.8023, 87.3231) centre (-65.859, 88.3215) ccw projected
  arc A41 (-60.3905, 85.4377) -> (-65.8023, 87.3231) centre (-65.3767, 79.8352) ccw projected
  arc A42 (-60.3905, 85.4377) -> (-59.2073, 85.3296) centre (-59.7257, 86.1847) ccw projected
  line L10 (-59.2073, 85.3296) -> (-48.9817, 91.5288) projected
  arc A43 (-48.9817, 91.5288) -> (-48.5003, 92.4053) centre (-49.5001, 92.3839) ccw projected
  arc A44 (-48.4958, 92.6994) -> (-48.5003, 92.4053) centre (-44.5012, 92.4909) ccw projected
  arc A45 (-48.4958, 92.6994) -> (-48.95, 93.5904) centre (-49.4944, 92.7516) ccw projected
  line L11 (-48.95, 93.5904) -> (-49.574, 93.9954) projected
  arc A46 (-49.574, 93.9954) -> (-50.1478, 94.1562) centre (-50.1185, 93.1567) ccw projected
  arc A47 (-52.021, 94.5252) -> (-50.1478, 94.1562) centre (-50.2742, 98.4544) ccw projected
  arc A48 (-52.021, 94.5252) -> (-53.0094, 94.4244) centre (-52.4272, 93.6114) ccw projected
  arc A49 (-65.771, 98.9569) -> (-53.0094, 94.4244) centre (-57.8128, 101.1319) ccw projected
  arc A50 (-65.771, 98.9569) -> (-66.4744, 99.6586) centre (-66.7356, 98.6933) ccw projected
  circle A51 centre (-65.3767, 52.702) radius 1.5 projected
  circle A52 centre (-57.0131, 57.3673) radius 1.3 projected
  circle A53 centre (-50.8767, 62.5) radius 5.25 projected
  circle A54 centre (-44.7404, 67.6327) radius 1.3 projected
  line L12 (-63.8767, 71.7112) -> (-63.8767, 57.4086) projected
  arc A55 (-63.8767, 57.4086) -> (-62.3169, 56.58) centre (-62.8767, 57.4086) ccw projected
  line L13 (-62.3169, 56.58) -> (-61.7354, 56.9729) projected
  arc A56 (-61.7354, 56.9729) -> (-61.2986, 57.7196) centre (-62.2953, 57.8015) ccw projected
  arc A57 (-59.5099, 60.8681) -> (-61.2986, 57.7196) centre (-57.0131, 57.3673) ccw projected
  arc A58 (-59.5099, 60.8681) -> (-59.0944, 61.7707) centre (-60.0905, 61.6823) ccw projected
  arc A59 (-51.4061, 70.733) -> (-59.0944, 61.7707) centre (-50.8767, 62.5) ccw projected
  arc A60 (-51.4061, 70.733) -> (-50.4921, 71.523) centre (-51.4703, 71.7309) ccw projected
  line L14 (-50.4921, 71.523) -> (-47.1705, 87.1482) projected
  arc A61 (-47.1705, 87.1482) -> (-48.6671, 88.2112) centre (-48.1487, 87.3561) ccw projected
  line L15 (-48.6671, 88.2112) -> (-58.3104, 82.365) projected
  arc A62 (-58.3494, 82.4556) -> (-58.3104, 82.365) centre (-57.4124, 82.805) ccw projected
  arc A63 (-63.1709, 72.667) -> (-58.3494, 82.4556) centre (-65.3767, 79.8352) ccw projected
  arc A64 (-63.1709, 72.667) -> (-63.8767, 71.7112) centre (-62.8767, 71.7112) ccw projected
  arc A65 (-69.9585, 53.9877) -> (-71.1263, 53.9531) centre (-70.5184, 53.1591) ccw projected
  arc A66 (-76.7449, 54.2911) -> (-71.1263, 53.9531) centre (-73.7404, 57.3673) ccw projected
  arc A67 (-76.7449, 54.2911) -> (-77.7067, 54.5405) centre (-77.4437, 53.5757) ccw projected
  arc A68 (-88.0944, 63.2293) -> (-77.7067, 54.5405) centre (-79.8767, 62.5) ccw projected
  arc A69 (-88.0944, 63.2293) -> (-88.5099, 64.1319) centre (-89.0905, 63.3177) ccw projected
  arc A70 (-89.8355, 69.6024) -> (-88.5099, 64.1319) centre (-86.0131, 67.6327) ccw projected
  arc A71 (-89.8355, 69.6024) -> (-90.0078, 70.7579) centre (-90.7244, 70.0604) ccw projected
  line L16 (-90.0078, 70.7579) -> (-90.9798, 71.7565) projected
  arc A72 (-90.9798, 71.7565) -> (-91.7931, 72.0544) centre (-91.6964, 71.059) ccw projected
  arc A73 (-92.8499, 77.9406) -> (-91.7931, 72.0544) centre (-92.0829, 75.0403) ccw projected
  arc A74 (-92.8499, 77.9406) -> (-92.1911, 78.5027) centre (-93.1056, 78.9074) ccw projected
  line L17 (-92.1911, 78.5027) -> (-91.6272, 79.7771) projected
  arc A75 (-91.6272, 79.7771) -> (-91.8676, 80.9205) centre (-92.5416, 80.1818) ccw projected
  arc A76 (-92.5278, 86.5104) -> (-91.8676, 80.9205) centre (-88.9691, 84.0968) ccw projected
  arc A77 (-92.5278, 86.5104) -> (-92.4523, 87.5011) centre (-93.3554, 87.0717) ccw projected
  arc A78 (-85.7359, 99.2608) -> (-92.4523, 87.5011) centre (-85.0015, 91.0436) ccw projected
  arc A79 (-85.7359, 99.2608) -> (-84.921, 99.8292) centre (-85.8249, 100.2569) ccw projected
  arc A80 (-79.7708, 102.1007) -> (-84.921, 99.8292) centre (-81.034, 97.9904) ccw projected
  arc A81 (-79.7708, 102.1007) -> (-78.6639, 102.4745) centre (-79.4771, 103.0566) ccw projected
  line L18 (-78.6639, 102.4745) -> (-77.8528, 103.6077) projected
  arc A82 (-77.8528, 103.6077) -> (-77.7034, 104.4608) centre (-78.6659, 104.1898) ccw projected
  arc A83 (-72.0965, 106.5412) -> (-77.7034, 104.4608) centre (-74.8156, 105.2737) ccw projected
  arc A84 (-72.0965, 106.5412) -> (-71.4268, 105.9921) centre (-71.1901, 106.9637) ccw projected
  line L19 (-71.4268, 105.9921) -> (-70.0728, 105.6623) projected
  arc A85 (-70.0728, 105.6623) -> (-68.99, 106.1009) centre (-69.8361, 106.6338) ccw projected
  arc A86 (-63.6047, 107.7386) -> (-68.99, 106.1009) centre (-65.3514, 103.8094) ccw projected
  arc A87 (-63.6047, 107.7386) -> (-62.6162, 107.8393) centre (-63.1984, 108.6523) ccw projected
  arc A88 (-49.8547, 103.3068) -> (-62.6162, 107.8393) centre (-57.8128, 101.1319) ccw projected
  arc A89 (-49.8547, 103.3068) -> (-49.1512, 102.6051) centre (-48.89, 103.5704) ccw projected
  arc A90 (-46.0508, 97.6465) -> (-49.1512, 102.6051) centre (-50.2742, 98.4544) ccw projected
  arc A91 (-46.0508, 97.6465) -> (-44.9551, 96.465) centre (-45.0686, 97.4586) ccw projected
  arc A92 (-43.2653, 88.6866) -> (-44.9551, 96.465) centre (-44.5012, 92.4909) ccw projected
  arc A93 (-43.2653, 88.6866) -> (-43.9344, 87.9435) centre (-42.9563, 87.7355) ccw projected
  line L20 (-43.9344, 87.9435) -> (-47.1214, 72.9516) projected
  arc A94 (-47.1214, 72.9516) -> (-45.8786, 71.7794) centre (-46.1433, 72.7437) ccw projected
  arc A95 (-42.2436, 64.1319) -> (-45.8786, 71.7794) centre (-44.7404, 67.6327) ccw projected
  arc A96 (-42.2436, 64.1319) -> (-42.659, 63.2293) centre (-41.663, 63.3177) ccw projected
  arc A97 (-53.0468, 54.5405) -> (-42.659, 63.2293) centre (-50.8767, 62.5) ccw projected
  arc A98 (-53.0468, 54.5405) -> (-54.0085, 54.2911) centre (-53.3098, 53.5757) ccw projected
  arc A99 (-59.6272, 53.9531) -> (-54.0085, 54.2911) centre (-57.0131, 57.3673) ccw projected
  arc A100 (-59.6272, 53.9531) -> (-60.795, 53.9877) centre (-60.2351, 53.1591) ccw projected
  line L21 (-60.795, 53.9877) -> (-61.9497, 53.2074) projected
  arc A101 (-61.9497, 53.2074) -> (-62.3865, 52.4596) centre (-61.3898, 52.3788) ccw projected
  arc A102 (-68.3669, 52.4596) -> (-62.3865, 52.4596) centre (-65.3767, 52.702) ccw projected
  arc A103 (-68.3669, 52.4596) -> (-68.8038, 53.2074) centre (-69.3637, 52.3788) ccw projected
  line L22 (-68.8038, 53.2074) -> (-69.9585, 53.9877) projected
  arc A104 (-63.1709, 72.667) -> (-58.3494, 82.4556) centre (-65.3767, 79.8352) ccw projected
  circle A105 centre (-65.3767, 79.8352) radius 5.25
  point P0 (0, 0)
  dimension "d6" = 10.5
  constraints: 1 centre point, 1 coincident
  measures "d6" diameter of A105
extrude "押し出し2" cut sketch "スケッチ2" against normal blind 0.6 contours A13 | A105